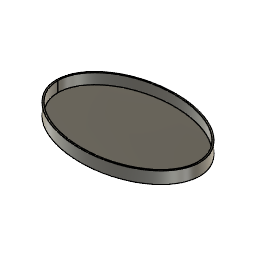
Sewing Dish Assembly (Autodesk Fusion 360 archive; units mm, degrees)
design "Dish"
part number: 2026-02-12-14-42-06-451
Autodesk Fusion 360 part; units mm, degrees
sketch "Sketch1" plane through (0, 0, 0) normal (0, 0, 1) x (1, 0, 0)
  ellipse E0 centre (0, 0) end of major axis (150, 0) minor radius 100
  line L0 (-150, 0) -> (150, 0) construction
  line L1 (0, -100) -> (0, 100) construction
  dimension "d1" = 200
  dimension "d2" = 300
  constraint coincident E0 L0.start
  constraint coincident E0 L0.end
  constraint coincident E0 L1.start
  constraint coincident E0 L1.end
  constraint coincident E0.centre origin
  constraint horizontal L0
  measures "d2" distance of E0
extrude "Extrude1" add sketch "Sketch1" along normal blind 25
shell "Shell1" thickness 3 removed faces 1 at (4.5867, 33.1249, 25)
